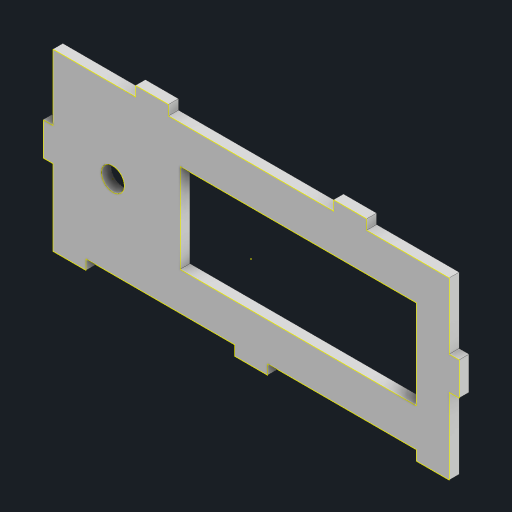
# Autodesk Inventor part: Front-panel
Saved by Autodesk Inventor 2023 (Build 270158000, 158)
## iProperties
Created: 2024-07-21
Part Number: Front-panel
Material: Generic
Document SubType Name: Modeling
Designer: Orsted
Density: 1 g/cm^3
Appearance: Default
Author: Orsted
Autodesk Inventor part; units mm, degrees
ref_plane "YZ Plane" through (0, 0, 0) normal (1, 0, 0) x (0, 1, 0)
ref_plane "XZ Plane" through (0, 0, 0) normal (0, 1, 0) x (-1, 0, 0)
ref_plane "XY Plane" through (0, 0, 0) normal (0, 0, 1) x (1, 0, 0)
sketch "Sketch1" plane through (0, 0, 0) normal (0, 0, 1) x (1, 0, 0)
  line L0 (60, -25) -> (-60, -25)
  line L1 (-60, -25) -> (-60, 25)
  line L2 (-60, 25) -> (60, 25)
  line L3 (60, 25) -> (60, -25)
  line L4 (60, -25) -> (-60, 25) construction
  line L5 (-60, -25) -> (60, 25) construction
  line L6 (50, -13.5) -> (-21.5, -13.5)
  line L7 (-21.5, -13.5) -> (-21.5, 13.5)
  line L8 (-21.5, 13.5) -> (50, 13.5)
  line L9 (50, 13.5) -> (50, -13.5)
  line L10 (50, -13.5) -> (-21.5, 13.5) construction
  line L11 (-21.5, -13.5) -> (50, 13.5) construction
  line L12 (-33.5, -13.1) -> (-52.2, -13.1)
  line L13 (-52.2, -13.1) -> (-52.2, 13.1)
  line L14 (-52.2, 13.1) -> (-33.5, 13.1)
  line L15 (-33.5, 13.1) -> (-33.5, -13.1)
  line L16 (-33.5, -13.1) -> (-52.2, 13.1) construction
  line L17 (-52.2, -13.1) -> (-33.5, 13.1) construction
  circle A0 centre (-41.9, 0) radius 3.5
  line L18 (-5, 28) -> (5, 28)
  line L19 (5, 28) -> (5, 25)
  line L20 (5, 25) -> (-5, 25)
  line L21 (-5, 25) -> (-5, 28)
  line L22 (-5, -25) -> (5, -25)
  line L23 (5, -25) -> (5, -28)
  line L24 (5, -28) -> (-5, -28)
  line L25 (-5, -28) -> (-5, -25)
  line L26 (-60, 28) -> (-50, 28)
  line L27 (-50, 28) -> (-50, 25)
  line L28 (-50, 25) -> (-60, 25)
  line L29 (-60, 25) -> (-60, 28)
  line L30 (50, 28) -> (60, 28)
  line L31 (60, 28) -> (60, 25)
  line L32 (60, 25) -> (50, 25)
  line L33 (50, 25) -> (50, 28)
  line L34 (-60, -25) -> (-50, -25)
  line L35 (-50, -25) -> (-50, -28)
  line L36 (-50, -28) -> (-60, -28)
  line L37 (-60, -28) -> (-60, -25)
  line L38 (50, -25) -> (60, -25)
  line L39 (60, -25) -> (60, -28)
  line L40 (60, -28) -> (50, -28)
  line L41 (50, -28) -> (50, -25)
  line L42 (-63, 5) -> (-60, 5)
  line L43 (-60, 5) -> (-60, -5)
  line L44 (-60, -5) -> (-63, -5)
  line L45 (-63, -5) -> (-63, 5)
  line L46 (63, -5) -> (60, -5)
  line L47 (60, -5) -> (60, 5)
  line L48 (60, 5) -> (63, 5)
  line L49 (63, 5) -> (63, -5)
  point P0 (0, 0)
  point P1 (14.25, 0)
  point P2 (-42.85, 0)
  point P3 (0, 25)
  point P4 (0, -25)
  point P5 (-60, 0)
  point P6 (60, 0)
  dimension "d0" = 120
  dimension "d1" = 50
  dimension "d2" = 27
  dimension "d3" = 71.5
  dimension "d4" = 10
  dimension "d6" = 18.7
  dimension "d7" = 26.2
  dimension "d8" = 7
  dimension "d9" = 8.4
  dimension "d10" = 12
  dimension "d11" = 10
  dimension "d12" = 3
  dimension "d13" = 10
  dimension "d14" = 3
  dimension "d15" = 10
  dimension "d16" = 3
  dimension "d17" = 10
  dimension "d18" = 3
  dimension "d19" = 10
  dimension "d20" = 3
  dimension "d21" = 10
  dimension "d22" = 3
  dimension "d23" = 3
  dimension "d24" = 10
  dimension "d25" = 3
  dimension "d26" = 10
  constraints: 100 end point, 22 parallel, 13 midpoint, 11 horizontal, 11 perpendicular, 2 horizontal alignment, 1 centre point
  measures "d0" distance of L1.end L2.end
  measures "d1" distance of L2.end L0.start
  measures "d2" distance between parallel lines of L6 L8
  measures "d3" distance of L7.end L8.end
  measures "d4" distance between parallel lines of L3 L9
  measures "d6" distance of L13.end L14.end
  measures "d7" distance of L12.end L13.end
  measures "d8" diameter of A0
  measures "d9" distance from line of L15 A0.centre
  measures "d10" distance between parallel lines of L7 L15
  measures "d11" distance of L19.end L20.end
  measures "d12" distance of L18.end L19.end
  measures "d13" distance of L23.end L24.end
  measures "d14" distance of L22.end L23.end
  measures "d15" distance of L1.end L27.end
  measures "d16" distance of L26.end L27.end
  measures "d17" distance of L2.end L32.end
  measures "d18" distance of L2.end L30.end
  measures "d19" distance of L35.end L36.end
  measures "d20" distance of L34.end L35.end
  measures "d21" distance of L39.end L40.end
  measures "d22" distance of L0.start L39.end
  measures "d23" distance of L43.end L44.end
  measures "d24" distance of L42.end L43.end
  measures "d25" distance of L47.end L48.end
  measures "d26" distance of L46.end L47.end
extrude "Extrusion1" add sketch "Sketch1" along normal blind 3 contours L39 L40 L41 L0 | L0 L1 L2 L3 | L3 L48 L49 L46 | L23 L24 L25 L0 | L2 L33 L30 L31 | L35 L36 L37 L0 | L2 L21 L18 L19 | L44 L45 L42 L1 | L2 L29 L26 L27 | L12 L13 L14 L15
sketch "Sketch2" plane through (0, 0, 3) normal (0, 0, 1) x (1, 0, 0)
  line L0 (-60, 28) -> (-60, 5) projected
  line L1 (-50, 28) -> (-60, 28) projected
  line L2 (-50, 25) -> (-50, 28) projected
  line L3 (-5, 25) -> (-50, 25) projected
  line L4 (60, 5) -> (60, 28) projected
  line L5 (60, 28) -> (50, 28) projected
  line L6 (50, 28) -> (50, 25) projected
  line L7 (50, 25) -> (5, 25) projected
  line L8 (5, 25) -> (5, 28) projected
  line L9 (5, 28) -> (-5, 28) projected
  line L10 (-5, 28) -> (-5, 25) projected
  line L11 (-60, 25) -> (60, 25)
  point P0 (0, 0)
  constraints: 3 point on line, 2 end point
extrude "Extrusion2" cut sketch "Sketch2" against normal through all
sketch "Sketch3" plane through (0, 0, 3) normal (0, 0, 1) x (1, 0, 0)
  line L0 (60, 25) -> (-60, 25) projected
  line L1 (-35, 28) -> (-25, 28)
  line L2 (-25, 28) -> (-25, 25)
  line L3 (-25, 25) -> (-35, 25)
  line L4 (-35, 25) -> (-35, 28)
  line L5 (25, 28) -> (35, 28)
  line L6 (35, 28) -> (35, 25)
  line L7 (35, 25) -> (25, 25)
  line L8 (25, 25) -> (25, 28)
  point P0 (0, 0)
  point P1 (-30, 25)
  point P2 (0, 25)
  point P3 (-30, 28)
  point P4 (30, 25)
  dimension "d31" = 120
  dimension "d32" = 10
  dimension "d33" = 3
  dimension "d34" = 10
  dimension "d35" = 3
  dimension "d36" = 30
  dimension "d37" = 30
  constraints: 16 end point, 4 midpoint, 4 parallel, 2 horizontal, 2 perpendicular, 2 point on line
  measures "d31" distance of L0.start L0.end
  measures "d32" distance of L2.end L3.end
  measures "d33" distance of L1.end L2.end
  measures "d34" distance of L6.end L7.end
  measures "d35" distance of L5.end L6.end
  measures "d36" horizontal distance of point (0, 25) point (-30, 28)
  measures "d37" distance of point (0, 25) point (30, 25)
extrude "Extrusion3" add sketch "Sketch3" against normal blind 3
sketch "Sketch4" plane through (0, 0, 3) normal (0, 0, 1) x (1, 0, 0)
  circle A0 centre (-41.9, 0) radius 3.5 projected
  line L0 (50, -13.5) -> (50, 13.5) projected
  line L1 (50, 13.5) -> (-21.5, 13.5) projected
  line L2 (-21.5, 13.5) -> (-21.5, -13.5) projected
  line L3 (-21.5, -13.5) -> (50, -13.5) projected
  line L4 (60, 5) -> (63, 5) projected
  line L5 (63, 5) -> (63, -5) projected
  line L6 (63, -5) -> (60, -5) projected
  line L7 (60, -5) -> (60, -28) projected
  line L8 (60, -28) -> (50, -28) projected
  line L9 (50, -28) -> (50, -25) projected
  line L10 (50, -25) -> (5, -25) projected
  line L11 (5, -25) -> (5, -28) projected
  line L12 (5, -28) -> (-5, -28) projected
  line L13 (-5, -28) -> (-5, -25) projected
  line L14 (-5, -25) -> (-50, -25) projected
  line L15 (-50, -25) -> (-50, -28) projected
  line L16 (-50, -28) -> (-60, -28) projected
  line L17 (-60, -28) -> (-60, -5) projected
  line L18 (-60, -5) -> (-63, -5) projected
  line L19 (-63, -5) -> (-63, 5) projected
  line L20 (-63, 5) -> (-60, 5) projected
  line L21 (-60, 5) -> (-60, 25) projected
  line L22 (-60, 25) -> (-35, 25) projected
  line L23 (-35, 25) -> (-35, 28) projected
  line L24 (-35, 28) -> (-25, 28) projected
  line L25 (-25, 28) -> (-25, 25) projected
  line L26 (-25, 25) -> (25, 25) projected
  line L27 (25, 25) -> (25, 28) projected
  line L28 (25, 28) -> (35, 28) projected
  line L29 (35, 28) -> (35, 25) projected
  line L30 (35, 25) -> (60, 25) projected
  line L31 (60, 25) -> (60, 5) projected
  point P0 (0, 0)
equation "\"d36\" = 0.25 * d31"
equation "\"d37\" = d36"
body "Solid1"
